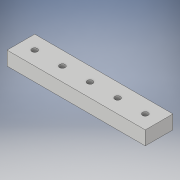
# Autodesk Inventor part: Linear_rail
Saved by Autodesk Inventor 2019 (Build 230136000, 136)
## iProperties
Created: 2021-06-02
Part Number: Linear_rail
Material: Generisch
Document SubType Name: Modeling
Designer: Bergi
Density: 1 g/cm^3
Appearance: Vorgabe
Author: Bergi
Autodesk Inventor part; units mm, degrees
ref_plane "YZ Plane" through (0, 0, 0) normal (1, 0, 0) x (0, 1, 0)
ref_plane "XZ Plane" through (0, 0, 0) normal (0, 1, 0) x (-1, 0, 0)
ref_plane "XY Plane" through (0, 0, 0) normal (0, 0, 1) x (1, 0, 0)
sketch "Skizze1" plane through (0, 0, 0) normal (0, 1, 0) x (-1, 0, 0)
  line L0 (-50, 10) -> (50, 10)
  line L1 (50, 10) -> (50, -10)
  line L2 (50, -10) -> (-50, -10)
  line L3 (-50, -10) -> (-50, 10)
  line L4 (-50, 10) -> (50, -10) construction
  line L5 (50, 10) -> (-50, -10) construction
  point P0 (0, 0)
  dimension "d0" = 100
  dimension "d1" = 20
  constraints: 12 end point, 2 midpoint, 2 parallel, 1 horizontal, 1 perpendicular
  measures "d0" distance of L1.end L2.end
  measures "d1" distance of L0.end L1.end
extrude "Extrusion1" add sketch "Skizze1" along normal blind 10
sketch "Skizze2" plane through (0, 10, 0) normal (0, 1, 0) x (1, 0, 0)
  line L0 (-70, 0) -> (70, 0) projected
  line L1 (-50, 10) -> (-50, -10) projected
  point P0 (0, 0)
  point P1 (-40, 0)
  point P2 (-20, 0)
  point P3 (0, 0)
  point P4 (20, 0)
  point P5 (40, 0)
  dimension "d4" = 10
  dimension "d7" = 20
  constraints: 1 horizontal, 1 point on line, 4 other
  measures "d4" distance from line of L1 point (-40, 0)
  measures "d7" distance of point (-40, 0) point (-20, 0)
hole "Bohrung1" at (-40, 10, 0) at (-20, 10, 0) at (0, 10, 0) at (20, 10, 0) at (40, 10, 0) direction (0, -1, 0) diameter 4 end through all
